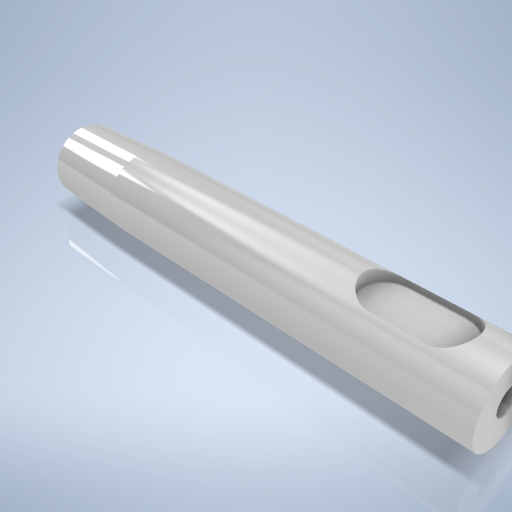
# Autodesk Inventor part: Welle
Saved by Autodesk Inventor 2024.2 (Build 282272000, 272)
## iProperties
Created: 2024-04-16
Part Number: Welle
Material: Aluminum 6061-AHC
Document SubType Name: Modeling
Designer: Fabri
Density: 2.7 g/cm^3
Appearance: Aluminium - dunkel
Author: Fabri
Autodesk Inventor part; units mm, degrees
ref_plane "YZ Plane" through (0, 0, 0) normal (1, 0, 0) x (0, 1, 0)
ref_plane "XZ Plane" through (0, 0, 0) normal (0, 1, 0) x (-1, 0, 0)
sketch "Skizze1" plane through (0, 0, 0) normal (0, 0, 1) x (1, 0, 0)
  line L0 (0, 0) -> (0, 4.5197)
  line L1 (0, 4.5197) -> (11, 5)
  line L2 (11, 5) -> (58, 5)
  line L3 (58, 5) -> (58, 0)
  line L4 (58, 0) -> (0, 0)
  dimension "d0" = 2.5
  dimension "d1" = 58
  dimension "d2" = 10
  dimension "d3" = 11
  constraints: 10 end point, 3 perpendicular, 1 vertical
  measures "d0" angle of L2 L1
  measures "d1" distance between parallel lines of L3 L0
  measures "d2" diameter of L2.end L4
  measures "d3" distance from line of L1.end L0
revolve "Umdrehung1" add sketch "Skizze1" angle 360 about axis through (58, 0, 0) along (-1, 0, 0)
ref_plane "Arbeitsebene1" through (0, 0, 5) normal (0, 0, 1) x (1, 0, 0)
sketch "Skizze2" plane through (0, 0, 5) normal (0, 0, 1) x (1, 0, 0)
  line L0 (58, 5) -> (58, -5) projected
  line L1 (0, 0) -> (78.1266, 0) construction
  line L2 (45.5, 0) -> (51.5, 0) construction
  line L3 (45.5, -3) -> (51.5, -3)
  line L4 (51.5, 3) -> (45.5, 3)
  arc A0 (45.5, 3) -> (45.5, -3) centre (45.5, 0) ccw
  arc A1 (51.5, -3) -> (51.5, 3) centre (51.5, 0) ccw
  point P0 (48.5, 0)
  point P1 (58, 0)
  point P2 (54.5, 0)
  point P3 (42.5, 0)
  dimension "d8" = 12
  dimension "d9" = 3.5
  dimension "d10" = 3
  constraints: 10 end point, 6 point on circle, 4 tangent, 2 centre point, 2 midpoint, 2 point on line, 1 horizontal, 1 horizontal alignment, 1 parallel, 1 other
  measures "d8" distance of point (54.5, 0) point (42.5, 0)
  measures "d9" distance from line of L0 point (54.5, 0)
  measures "d10" radius of A1
extrude "Extrusion1" cut sketch "Skizze2" against normal blind 1.8
sketch "Skizze3" plane through (0, 0, 0) normal (-1, 0, 0) x (0, 0, 1)
  circle A0 centre (0, 0) radius 4.5197 projected
  constraints: 1 coincident
hole "Bohrung1" at (0, 0, 0) direction (1, 0, 0) diameter 3.242 depth 58 counterbore diameter 6 counterbore depth 2.5 thread size "M4x0.7" class "6H" standard "ISO Metric profile"
